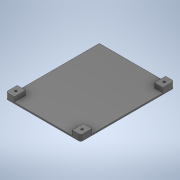
# Autodesk Inventor part: FLC_Holder
Saved by Autodesk Inventor 2020 (Build 240168000, 168)
## iProperties
Created: 2020-04-23
Part Number: FLC_Holder
Material: Типовые
Document SubType Name: Modeling
Designer: Михаил
Density: 1 g/cm^3
Appearance: По умолчанию
Author: Михаил
Autodesk Inventor part; units mm, degrees
ref_plane "YZ Plane" through (0, 0, 0) normal (1, 0, 0) x (0, 1, 0)
ref_plane "XZ Plane" through (0, 0, 0) normal (0, 1, 0) x (-1, 0, 0)
ref_plane "XY Plane" through (0, 0, 0) normal (0, 0, 1) x (1, 0, 0)
sketch "Эскиз1" plane through (0, 0, 0) normal (0, 1, 0) x (-1, 0, 0)
  line L0 (0, 0) -> (80, 0)
  line L1 (80, 0) -> (80, -100)
  line L2 (80, -100) -> (0, -100)
  line L3 (0, -100) -> (0, 0)
  dimension "d0" = 80
  dimension "d1" = 100
  constraints: 8 end point, 2 parallel, 1 horizontal, 1 perpendicular
  measures "d0" distance of L1.end L2.end
  measures "d1" distance of L0.end L1.end
extrude "Выдавливание1" add sketch "Эскиз1" along normal blind 1.5
sketch "Эскиз2" plane through (0, 1.5, 0) normal (0, 1, 0) x (1, 0, 0)
  circle A0 centre (-4.5, 94) radius 1.25
  circle A1 centre (-4.5, 6) radius 1.25
  circle A2 centre (-75.5, 6) radius 1.25
  line L0 (0, 0) -> (0, 100) projected
  line L1 (0, 100) -> (-80, 100) projected
  line L2 (-80, 0) -> (0, 0) projected
  line L3 (-80, 100) -> (-80, 0) projected
  dimension "d4" = 2.5
  dimension "d5" = 2.5
  dimension "d6" = 2.5
  dimension "d7" = 4.5
  dimension "d8" = 6
  dimension "d9" = 4.5
  dimension "d10" = 6
  dimension "d11" = 4.5
  dimension "d12" = 6
  constraints: 3 centre point
  measures "d4" diameter of A0
  measures "d5" diameter of A1
  measures "d6" diameter of A2
  measures "d7" distance from line of L0 A0.centre
  measures "d8" distance from line of L1 A0.centre
  measures "d9" distance from line of L0 A1.centre
  measures "d10" distance from line of A1.centre L2
  measures "d11" distance from line of L3 A2.centre
  measures "d12" distance from line of A2.centre L2
sketch "Эскиз3" plane through (0, 1.5, 0) normal (0, 1, 0) x (1, 0, 0)
  line L0 (-80, 0) -> (0, 0) projected
  line L1 (0, 0) -> (-9, 0)
  line L2 (-9, 0) -> (-9, 12)
  line L3 (-9, 12) -> (0, 12)
  line L4 (0, 12) -> (0, 0)
  line L5 (0, 100) -> (-80, 100) projected
  line L6 (0, 100) -> (-9, 100)
  line L7 (-9, 100) -> (-9, 88)
  line L8 (-9, 88) -> (0, 88)
  line L9 (0, 88) -> (0, 100)
  line L10 (-80, 100) -> (-80, 0) projected
  line L11 (-80, 0) -> (-71, 0)
  line L12 (-71, 0) -> (-71, 12)
  line L13 (-71, 12) -> (-80, 12)
  line L14 (-80, 12) -> (-80, 0)
  dimension "d13" = 9
  dimension "d14" = 12
  dimension "d15" = 9
  dimension "d16" = 12
  dimension "d17" = 9
  dimension "d18" = 12
  constraints: 24 end point, 6 parallel, 3 horizontal, 3 perpendicular
  measures "d13" distance of L2.end L3.end
  measures "d14" distance of L1.end L2.end
  measures "d15" distance of L8.end L7.end
  measures "d16" distance of L7.end L6.end
  measures "d17" distance of L13.end L12.end
  measures "d18" distance of L12.end L11.end
extrude "Выдавливание2" add sketch "Эскиз3" along normal blind 5
extrude "Выдавливание3" cut sketch "Эскиз2" along normal blind 5 contours A0 | A1 | A2
fillet "Сопряжение1" radius 2 3 edges at (0, 3.25, 0) (0, 3.25, -100) (-80, 3.25, 0)
